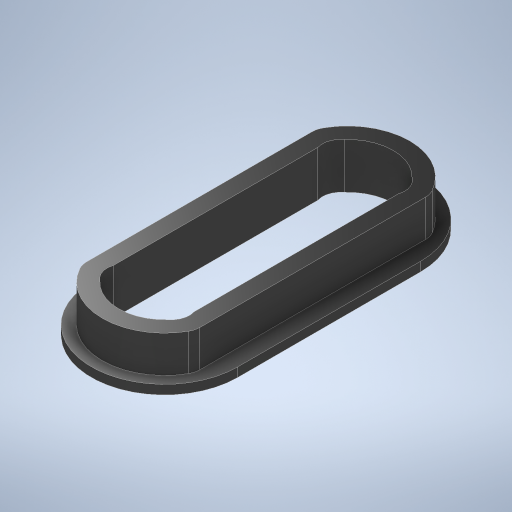
# Autodesk Inventor part: SliderProtectionFrame
Saved by Autodesk Inventor 2024.2 (Build 282272000, 272)
## iProperties
Created: 2024-06-04
Part Number: SliderProtectionFrame
Material: Aluminum 7075
Document SubType Name: Modeling
Designer: Masato Kubotera
Density: 2.81 g/cm^3
Appearance: Glossy - Black
Mass: 2.25762 g
Surface Area: 13.1383 cm^2
Volume: 0.803422 cm^3
Author: Masato Kubotera
Autodesk Inventor part; units mm, degrees
ref_plane "YZ Plane" through (0, 0, 0) normal (1, 0, 0) x (0, 1, 0)
ref_plane "XZ Plane" through (0, 0, 0) normal (0, 1, 0) x (-1, 0, 0)
ref_plane "XY Plane" through (0, 0, 0) normal (0, 0, 1) x (1, 0, 0)
sketch "Sketch1" plane through (0, 0, 0) normal (0, 1, 0) x (-1, 0, 0)
  line L0 (6.25, 12.8036) -> (6.25, -12.8036) construction
  arc A0 (6.25, 12.8036) -> (-6.25, 12.8036) centre (0, 10) ccw construction
  arc A1 (4.4, 12.3749) -> (-4.4, 12.3749) centre (0, 10) ccw
  line L1 (4.4, 12.3749) -> (4.4, -12.3749)
  line L2 (-6.25, 12.8036) -> (-6.25, -12.8036) construction
  arc A2 (-6.25, -12.8036) -> (6.25, -12.8036) centre (0, -10) ccw construction
  arc A3 (-4.4, -12.3749) -> (4.4, -12.3749) centre (0, -10) ccw
  line L3 (-8, 0) -> (8, 0) construction
  circle A4 centre (0, -10) radius 7 construction
  arc A5 (3.6981, -13.3651) -> (4.4, -11.1611) centre (2.4943, -11.768) ccw
  line L4 (-4.4, 12.3749) -> (-4.4, -12.3749)
  arc A6 (-4.4, -11.1611) -> (-3.6981, -13.3651) centre (-2.4943, -11.768) ccw
  arc A7 (4.4, 11.1611) -> (3.6981, 13.3651) centre (2.4943, 11.768) ccw
  arc A8 (-3.6981, 13.3651) -> (-4.4, 11.1611) centre (-2.4943, 11.768) ccw
  arc A9 (-8, -10) -> (8, -10) centre (0, -10) ccw
  line L5 (8, -10) -> (8, 10)
  arc A10 (8, 10) -> (-8, 10) centre (0, 10) ccw
  line L6 (0, 10) -> (0, -10)
  line L7 (6.2, -12.7928) -> (6.2, 12.7928)
  arc A11 (6.2, 12.7928) -> (-6.2, 12.7928) centre (0, 10) ccw
  line L8 (-6.2, -12.7928) -> (-6.2, 12.7928)
  arc A12 (-6.2, -12.7928) -> (6.2, -12.7928) centre (0, -10) ccw
  line L9 (-8, -10) -> (-8, 10)
  point P0 (0, 0)
  point P1 (0, 0)
  point P2 (-3.6981, -13.3651)
  point P3 (4.4, 11.1611)
  point P4 (-6.2, -12.7928)
  dimension "d5" = 12.5
  dimension "d0" = 14
  dimension "d1" = 2
  dimension "d2" = 1
  dimension "d3" = 20
  dimension "d4" = 8.8
  dimension "d7" = 1.85
  dimension "d8" = 5
  dimension "d14" = 0.05
  dimension "d15" = 0.05
  constraints: 28 point on circle, 16 end point, 14 symmetric about line, 13 centre point, 4 coincident, 4 point on line, 3 midpoint, 3 vertical, 2 parallel, 1 concentric, 1 tangent, 15 other
  measures "d0" diameter of A4
  measures "d1" radius of A5
  measures "d2" radial gap between concentric circles of A9 A4
  measures "d3" distance of L6.start L6.end
  measures "d4" distance between parallel lines of L4 L1
  measures "d7" radial gap between concentric circles of A1 A0
  measures "d8" radius of A1
  measures "d15" radial gap between concentric circles of A2 A12
extrude "Extrusion1" add sketch "Sketch1" along normal blind 5 contours A12 L8 A11 L7
extrude "Extrusion2" add sketch "Sketch1" along normal blind 1 contours L9 A10 L5 A9
fillet "Fillet1" radius 2 4 edges at (6.2, 3, 12.7928) (6.2, 3, -12.7928) (-6.2, 3, -12.7928) (-6.2, 3, 12.7928)
equation "\"d7\" = -0.5 * d4 + 0.5 * d5"
equation "\"d15\" = d14"
body "Solid1"
